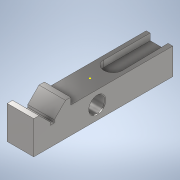
# Autodesk Inventor part: 5-压铁
Saved by Autodesk Inventor 2022 (Build 260153000, 153)
## iProperties
Created: 2023-01-08
Part Number: 5-压铁
Material: 不锈钢
Document SubType Name: Modeling
Designer: Lzy18
Density: 8 g/cm^3
Appearance: 半抛光
Author: Lzy18
Autodesk Inventor part; units mm, degrees
ref_plane "YZ Plane" through (0, 0, 0) normal (1, 0, 0) x (0, 1, 0)
ref_plane "XY Plane" through (0, 0, 0) normal (0, 0, 1) x (1, 0, 0)
sketch "草图1" plane through (0, 0, 0) normal (0, 1, 0) x (-1, 0, 0)
  line L0 (10, -52.5) -> (-10, -52.5)
  line L1 (-10, -52.5) -> (-10, 52.5)
  line L2 (-10, 52.5) -> (10, 52.5)
  line L3 (10, 52.5) -> (10, -52.5)
  line L4 (10, -52.5) -> (-10, 52.5) construction
  line L5 (-10, -52.5) -> (10, 52.5) construction
  point P0 (0, 0)
  dimension "d0" = 20
  dimension "d1" = 105
  constraints: 12 end point, 2 midpoint, 2 parallel, 1 horizontal, 1 perpendicular
  measures "d0" distance of L1.end L2.end
  measures "d1" distance of L0.end L1.end
extrude "拉伸1" add sketch "草图1" along normal blind 25
sketch "草图3" plane through (0, 25, 0) normal (0, 1, 0) x (1, 0, 0)
  line L0 (10, -52.5) -> (10, 52.5) projected
  line L1 (10, 52.5) -> (-10, 52.5) projected
  line L2 (-10, 52.5) -> (-10, -52.5) projected
  line L3 (-10, 52.5) -> (-10, -52.5) projected
  line L4 (-10, -52.5) -> (10, -52.5) projected
  line L5 (10, -52.5) -> (10, 52.5) projected
  line L6 (-10, 52.5) -> (-10, -28.5) projected
  line L7 (-10, -24.5) -> (10, -24.5)
  line L8 (10, -52.5) -> (10, 52.5) projected
  line L9 (10, 52.5) -> (-10, 52.5) projected
  line L10 (-10, -52.5) -> (10, -52.5) projected
  point P0 (0, 0)
  point P1 (10, -28.5)
  point P2 (10, -48.5)
  dimension "d12" = 28
  constraints: 2 end point, 2 point on line, 1 perpendicular
  measures "d12" distance between parallel lines of L4 L7
extrude "拉伸3" cut sketch "草图3" against normal blind 5 contours L7 L2 L1 L0
sketch "草图4" plane through (0, 20, 0) normal (0, 1, 0) x (1, 0, 0)
  point P0 (0, 0)
sketch "草图6" plane through (0, 0, 0) normal (1, 0, 0) x (0, 1, 0)
  line L0 (0, -52.5) -> (20, -52.5) projected
  line L1 (0, -52.5) -> (0, 52.5) projected
  circle A0 centre (10, 4.5) radius 6
  point P0 (0, 0)
  point P1 (15, -52.5)
  dimension "d18" = 57
  dimension "d19" = 10
  dimension "d20" = 12
  constraints: 1 centre point, 1 coincident
  measures "d18" distance from line of L0 point (10, 4.5)
  measures "d19" distance from line of L1 point (10, 4.5)
  measures "d20" diameter of A0
extrude "拉伸5" cut sketch "草图6" along normal mid plane 19
ref_plane "工作平面1" through (0, 10, 0) normal (0, 1, 0) x (-1, 0, 0)
sketch "草图8" plane through (0, 10, 0) normal (0, 1, 0) x (-1, 0, 0)
  line L0 (10, 52.5) -> (-10, 52.5) projected
  line L1 (10, -52.5) -> (10, 52.5) projected
  line L2 (-10, -52.5) -> (10, -52.5) projected
  line L3 (-10, 52.5) -> (-10, -52.5) projected
  line L4 (9.5, -1.5) -> (9.5, 10.5) projected
  line L5 (-9.5, 10.5) -> (-9.5, -1.5) projected
  line L6 (9.5, -1.5) -> (9.5, 10.5) projected
  line L7 (9.5, 4.5) -> (10, 4.5)
  line L8 (10, -52.5) -> (10, 52.5) projected
  line L9 (9.5, -1.5) -> (10, -2)
  line L10 (10, -2) -> (10, 4.5)
  line L11 (9.5, 4.5) -> (9.5, -1.5)
  line L12 (10, 4.5) -> (-10, 4.5)
  line L13 (-10, 52.5) -> (-10, -52.5) projected
  point P0 (0, 0)
  dimension "d24" = 135
  constraints: 10 end point, 3 point on line, 2 collinear, 2 perpendicular, 1 midpoint
  measures "d24" angle of L4 L9
revolve "旋转1" cut sketch "草图8" angle 360 about axis through (-10, 10, 4.5) along (1, 0, 0) contours L1 L9 L4 L7
mirror "镜像1" about plane through (0, 0, 0) normal (1, 0, 0) of "旋转1"
sketch "草图9" plane through (0, 0, 0) normal (1, 0, 0) x (0, 1, 0)
  line L0 (0, -52.5) -> (20, -52.5) projected
  line L1 (25, 24.5) -> (25, 52.5) projected
  line L2 (14.5, 38.5) -> (31.5646, 38.5)
  line L3 (14.5, 38.5) -> (14.5, 37)
  line L4 (14.5, 37) -> (16.5, 37)
  line L5 (16.5, 37) -> (25, 28.5)
  line L6 (25, 28.5) -> (25, 38.5)
  line L7 (25, 52.5) -> (25, 24.5)
  line L8 (14.5, 40) -> (16.5, 40)
  line L9 (16.5, 40) -> (25, 48.5)
  line L10 (14.5, 40) -> (14.5, 38.5)
  point P0 (0, 0)
  point P1 (15, -52.5)
  dimension "d26" = 91
  dimension "d27" = 10.5
  dimension "d28" = 1.5
  dimension "d29" = 2
  dimension "d30" = 45
  constraints: 18 end point, 5 symmetric about line, 3 point on line, 2 vertical, 1 horizontal, 1 midpoint, 1 perpendicular
  measures "d26" distance from line of L0 L2.start
  measures "d27" distance from line of L1 L2.start
  measures "d28" distance of L2.start L3.end
  measures "d29" distance of L3.end L4.end
  measures "d30" angle of L2 L5
extrude "拉伸6" cut sketch "草图9" along normal through all both and the other way through all
sketch "草图10" plane through (0, 20, 0) normal (0, 1, 0) x (1, 0, 0)
  line L0 (-10, 52.5) -> (-10, -52.5) projected
  line L1 (-10, 17.5) -> (10, 17.5)
  line L2 (10, -52.5) -> (10, 52.5) projected
  line L3 (-10, 52.5) -> (10, 52.5) projected
  circle A0 centre (0, 17.5) radius 7
  line L4 (-7, 17.5) -> (-7, 52.5)
  line L5 (10, 52.5) -> (-10, 52.5) projected
  line L6 (7, 17.5) -> (6.4266, 52.5)
  point P0 (0, 0)
  point P1 (6.9962, 17.7293)
  dimension "d33" = 35
  dimension "d34" = 14
  constraints: 6 end point, 6 point on line, 2 point on circle, 1 centre point, 1 horizontal, 1 midpoint, 1 vertical
  measures "d33" distance between parallel lines of L3 L1
  measures "d34" diameter of A0
extrude "拉伸7" cut sketch "草图10" against normal blind 5 contours L3 L6 L1 L4 | L1 A0
